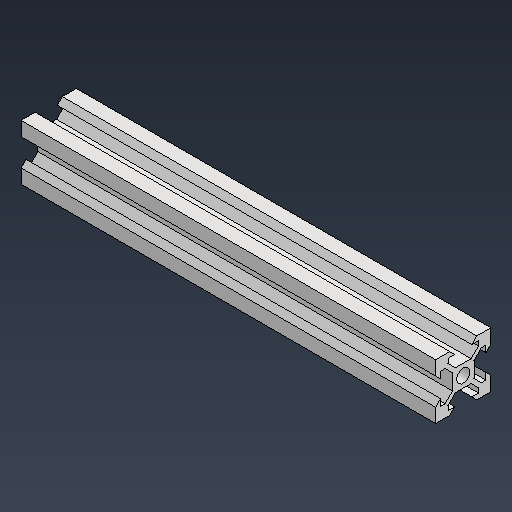
# Autodesk Inventor part: 2020
Saved by Autodesk Inventor 2026.2 (Build 302298010, 298A)
## iProperties
Created: 2026-06-05
Part Number: 2020
Material: Generic
Document SubType Name: Modeling
Designer: szymo
Density: 1 g/cm^3
Appearance: Default
Author: szymo
Autodesk Inventor part; units mm, degrees
ref_plane "YZ Plane" through (0, 0, 0) normal (1, 0, 0) x (0, 1, 0)
ref_plane "XZ Plane" through (0, 0, 0) normal (0, 1, 0) x (-1, 0, 0)
ref_plane "XY Plane" through (0, 0, 0) normal (0, 0, 1) x (1, 0, 0)
sketch "Sketch1" plane through (0, 0, 0) normal (1, 0, 0) x (0, 1, 0)
  line L0 (-10, -10) -> (10, -10)
  line L1 (10, -10) -> (10, 10)
  line L2 (10, 10) -> (-10, 10)
  line L3 (-10, 10) -> (-10, -10)
  line L4 (-10, -10) -> (10, 10) construction
  line L5 (10, -10) -> (-10, 10) construction
  line L6 (10, 4.9) -> (8.2, 3.1)
  line L7 (8.2, 3.1) -> (8.2, 5.4993)
  line L8 (8.2, 5.4993) -> (6.56, 5.4993)
  line L9 (6.56, 5.4993) -> (3.9007, 2.84)
  line L10 (3.9007, -2.84) -> (6.56, -5.4993)
  line L11 (6.56, -5.4993) -> (8.2, -5.4993)
  line L12 (8.2, -5.4993) -> (8.2, -3.1)
  line L13 (8.2, -3.1) -> (10, -4.9)
  circle A0 centre (0, 0) radius 2.4
  line L14 (3.9007, 2.84) -> (3.9007, -2.84)
  line L15 (3.9007, 0) -> (0, 0) construction
  line L16 (5.4993, 6.56) -> (5.4993, 8.2)
  line L17 (2.84, 3.9007) -> (5.4993, 6.56)
  line L18 (-2.84, 3.9007) -> (2.84, 3.9007)
  line L19 (-5.4993, 6.56) -> (-2.84, 3.9007)
  line L20 (-5.4993, 8.2) -> (-5.4993, 6.56)
  line L21 (-3.1, 8.2) -> (-5.4993, 8.2)
  line L22 (-4.9, 10) -> (-3.1, 8.2)
  line L23 (3.1, 8.2) -> (4.9, 10)
  line L24 (5.4993, 8.2) -> (3.1, 8.2)
  line L25 (-6.56, 5.4993) -> (-8.2, 5.4993)
  line L26 (-3.9007, 2.84) -> (-6.56, 5.4993)
  line L27 (-3.9007, -2.84) -> (-3.9007, 2.84)
  line L28 (-6.56, -5.4993) -> (-3.9007, -2.84)
  line L29 (-8.2, -5.4993) -> (-6.56, -5.4993)
  line L30 (-8.2, -3.1) -> (-8.2, -5.4993)
  line L31 (-10, -4.9) -> (-8.2, -3.1)
  line L32 (-8.2, 3.1) -> (-10, 4.9)
  line L33 (-8.2, 5.4993) -> (-8.2, 3.1)
  line L34 (-5.4993, -6.56) -> (-5.4993, -8.2)
  line L35 (-2.84, -3.9007) -> (-5.4993, -6.56)
  line L36 (2.84, -3.9007) -> (-2.84, -3.9007)
  line L37 (5.4993, -6.56) -> (2.84, -3.9007)
  line L38 (5.4993, -8.2) -> (5.4993, -6.56)
  line L39 (3.1, -8.2) -> (5.4993, -8.2)
  line L40 (4.9, -10) -> (3.1, -8.2)
  line L41 (-3.1, -8.2) -> (-4.9, -10)
  line L42 (-5.4993, -8.2) -> (-3.1, -8.2)
  point P0 (0, 3.9007)
  point P1 (-3.9007, 0)
  point P2 (0, -3.9007)
  dimension "d0" = 20
  dimension "d1" = 20
  dimension "d2" = 45
  dimension "d3" = 45
  dimension "d4" = 1.8
  dimension "d5" = 1.8
  dimension "d6" = 4.8
  dimension "d7" = 1.64
  dimension "d8" = 1.64
  dimension "d11" = 5.68
  dimension "d12" = 3.1
  dimension "d13" = 3.1
  dimension "d16" = 360
  dimension "d18" = 1.5
  dimension "d19" = 2.3993
  dimension "d20" = 2.3993
  constraints: 86 end point, 4 parallel, 3 horizontal, 3 midpoint, 3 perpendicular, 2 point on line, 1 centre point, 1 coincident, 1 vertical, 81 other
  measures "d0" distance of L2.end L1.end
  measures "d1" distance of L1.end L0.end
  measures "d2" angle of L1 L6
  measures "d3" angle of L1 L13
  measures "d4" distance between parallel lines of L1 L7
  measures "d5" distance between parallel lines of L1 L12
  measures "d6" diameter of A0
  measures "d7" distance of L7.end L8.end
  measures "d8" distance of L10.end L11.end
  measures "d11" distance of L9.end L10.start
  measures "d12" vertical distance of L15.end L6.end
  measures "d13" vertical distance of point (0, 0) L12.end
  measures "d18" distance between parallel lines of L17 L9
  measures "d19" distance of L6.end L7.end
  measures "d20" distance of L11.end L12.end
extrude "Extrusion1" add sketch "Sketch1" along normal blind 150 contours L3 L31 L30 L29 L28 L27 L26 L25 L33 L32 L2 L22 L21 L20 L19 L18 L17 L16 L24 L23 L1 L6 L7 L8 L9 L14 L10 L11 L12 L13 L0 L40 L39 L38 L37 L36 L35 L34 L42 L41
equation "\"d3\" = d2"
equation "\"d5\" = d4"
equation "\"d8\" = d7"
equation "\"d13\" = d12"
equation "\"d19\" = d20"
body "Solid1"
